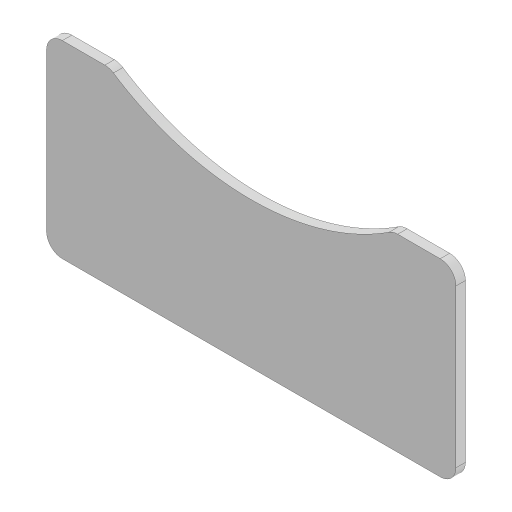
# Autodesk Inventor part: Base plate
Saved by Autodesk Inventor 2024 (Build 280153000, 153)
## iProperties
Created: 2025-04-26
Part Number: Base plate
Material: Generic
Document SubType Name: Modeling
Designer: Binara
Density: 1 g/cm^3
Appearance: Default
Author: Binara
Autodesk Inventor part; units mm, degrees
ref_plane "YZ Plane" through (0, 0, 0) normal (1, 0, 0) x (0, 1, 0)
ref_plane "XZ Plane" through (0, 0, 0) normal (0, 1, 0) x (-1, 0, 0)
ref_plane "XY Plane" through (0, 0, 0) normal (0, 0, 1) x (1, 0, 0)
sketch "Sketch1" plane through (0, 0, 0) normal (0, 0, 1) x (1, 0, 0)
  line L0 (-65, -30) -> (65, -30)
  line L1 (65, -30) -> (65, 30)
  line L2 (65, 30) -> (-65, 30)
  line L3 (-65, 30) -> (-65, -30)
  line L4 (-65, -30) -> (65, 30) construction
  line L5 (65, -30) -> (-65, 30) construction
  arc A0 (-45, 30) -> (45, 30) centre (0, 96.6789) ccw
  point P0 (0, 0)
  dimension "d0" = 130
  dimension "d1" = 60
  dimension "d5" = 20
  dimension "d6" = 20
  constraints: 12 end point, 2 midpoint, 2 parallel, 2 point on circle, 2 point on line, 1 centre point, 1 horizontal, 1 perpendicular
  measures "d0" distance of L2.end L1.end
  measures "d1" distance of L1.end L0.end
  measures "d5" distance from line of L1 A0.end
  measures "d6" distance from line of L3 A0.start
extrude "Extrusion1" add sketch "Sketch1" along normal blind 3 contours L3 L2 A0 L1 L0
fillet "Fillet1" radius 5 6 edges at (65, 30, 1.5) (65, -30, 1.5) (-65, -30, 1.5) (-65, 30, 1.5) (45, 30, 1.5) (-45, 30, 1.5)
equation "\"d6\" = d5"
body "Solid1"
